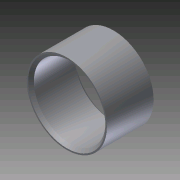
# Autodesk Inventor part: Metal Cylinder Seal 1764
Saved by Autodesk Inventor 2011 (Build 150239000, 239)
## iProperties
Created: 2010-01-18
Part Number: Metal Cylinder Seal 1764
Document SubType Name: Modeling
Designer: wbridges
Density: 1 g/cm^3
Author: wbridges
Autodesk Inventor part; units mm, degrees
ref_plane "YZ Plane" through (0, 0, 0) normal (1, 0, 0) x (0, 1, 0)
ref_plane "XZ Plane" through (0, 0, 0) normal (0, 1, 0) x (-1, 0, 0)
ref_plane "XY Plane" through (0, 0, 0) normal (0, 0, 1) x (1, 0, 0)
sketch "Sketch1" plane through (0, 0, 0) normal (0, 0, 1) x (1, 0, 0)
  circle A0 centre (0, 0) radius 15.875
  circle A1 centre (0, 0) radius 17.78
  dimension "d0" = 1.905
  dimension "d1" = 31.75
  constraints: 2 centre point, 2 coincident
  measures "d0" radial gap between concentric circles of A0 A1
  measures "d1" diameter of A0
extrude "Extrusion1" add sketch "Sketch1" along normal blind 20.701
chamfer "Chamfer1" distance 1.27 angle 45 2 edges at (-15.875, 0, 20.701) (-15.875, 0, 0)
body "Solid1"
